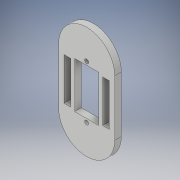
# Autodesk Inventor part: soporte servo base
Saved by Autodesk Inventor 2019 (Build 230136000, 136)
## iProperties
Created: 2020-02-10
Part Number: soporte servo base
Material: Generic
Document SubType Name: Modeling
Designer: jacqu
Density: 1 g/cm^3
Appearance: Default
base_servo: 12.000 mm
altura_servo: 23.000 mm
agujero_servo: 2.000 mm
distancia_agujero_servo: 1.750 mm
Author: jacqu
Autodesk Inventor part; units mm, degrees
ref_plane "YZ Plane" through (0, 0, 0) normal (1, 0, 0) x (0, 1, 0)
ref_plane "XZ Plane" through (0, 0, 0) normal (0, 1, 0) x (-1, 0, 0)
ref_plane "XY Plane" through (0, 0, 0) normal (0, 0, 1) x (1, 0, 0)
sketch "Sketch1" plane through (0, 0, 0) normal (0, 0, 1) x (1, 0, 0)
  line L0 (0, 0) -> (12, 0)
  line L1 (12, 0) -> (12, 23)
  line L2 (12, 23) -> (0, 23)
  line L3 (0, 23) -> (0, 0)
  line L4 (-8, -2.5) -> (-8, 25.5)
  line L5 (20, 25.5) -> (20, -2.5)
  arc A0 (20, 25.5) -> (-8, 25.5) centre (6, 25.5) ccw
  arc A1 (-8, -2.5) -> (20, -2.5) centre (6, -2.5) ccw
  dimension "base_servo" = 12
  dimension "altura_servo" = 23
  dimension "d2" = 8
  dimension "d3" = 8
  dimension "d4" = 28
  dimension "d5" = 28
  dimension "d9" = 2.5
  constraints: 12 end point, 4 point on circle, 3 tangent, 2 centre point, 2 parallel, 2 vertical, 1 horizontal, 1 perpendicular
  measures "base_servo" distance of L2.end L1.end
  measures "altura_servo" distance of L1.end L0.end
  measures "d2" distance between parallel lines of L4 L3
  measures "d3" distance between parallel lines of L5 L1
  measures "d4" distance of L4.start L4.end
  measures "d5" distance of L5.start L5.end
  measures "d9" distance from line of L0 A1.centre
extrude "Extrusion1" add sketch "Sketch1" along normal blind 3.3
sketch "Sketch2" plane through (0, 0, 3.3) normal (0, 0, 1) x (1, 0, 0)
  line L0 (14, 22) -> (17.3, 22)
  line L1 (17.3, 22) -> (17.3, 1)
  line L2 (17.3, 1) -> (14, 1)
  line L3 (14, 1) -> (14, 22)
  line L4 (-5.3, 22) -> (-2, 22)
  line L5 (-2, 22) -> (-2, 1)
  line L6 (-2, 1) -> (-5.3, 1)
  line L7 (-5.3, 1) -> (-5.3, 22)
  line L8 (0, 0) -> (0, 23) projected
  line L9 (12, 23) -> (12, 0) projected
  dimension "d12" = 3.3
  dimension "d13" = 3.3
  dimension "d14" = 21
  dimension "d16" = 1
  dimension "d17" = 2
  dimension "d18" = 2
  constraints: 16 end point, 4 parallel, 2 horizontal, 2 perpendicular, 2 point on line
  measures "d12" distance of L4.start L4.end
  measures "d13" distance of L0.start L0.end
  measures "d14" distance of L6.end L4.start
  measures "d16" distance from line of L8.end L4
  measures "d17" distance between parallel lines of L8 L5
  measures "d18" distance between parallel lines of L9 L3
extrude "Extrusion2" cut sketch "Sketch2" against normal blind 3.3
sketch "Sketch3" plane through (0, 0, 3.3) normal (0, 0, 1) x (1, 0, 0)
  circle A0 centre (6, 24.75) radius 1
  line L0 (0, 23) -> (12, 23) projected
  circle A1 centre (6, -1.75) radius 1
  line L1 (12, 0) -> (0, 0) projected
  dimension "agujero_servo" = 2
  dimension "distancia_agujero_servo" = 1.75
  dimension "d23" = 6
  dimension "d24" = 6
  dimension "d25" = 1.75
  constraints: 2 centre point, 1 equal radius
  measures "agujero_servo" diameter of A0
  measures "distancia_agujero_servo" distance from line of L0 A0.centre
  measures "d23" horizontal distance of A0.centre L1.end
  measures "d24" horizontal distance of L1.end A1.centre
  measures "d25" distance from line of L1 A1.centre
extrude "Extrusion3" cut sketch "Sketch3" against normal blind 3.3
equation "\"d3\" = d2"
equation "\"d5\" = d4"
equation "\"d9\" = 0.5 * d4 - 0.5 * altura_servo"
equation "\"d10\" = d12"
equation "\"d13\" = d12"
equation "\"d16\" = 0.5 * altura_servo - 0.5 * d14"
equation "\"d18\" = d17"
equation "\"d19\" = d12"
equation "\"d23\" = 0.5 * base_servo"
equation "\"d24\" = 0.5 * base_servo"
equation "\"d25\" = distancia_agujero_servo"
body "Solid1"
